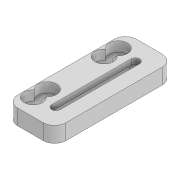
# Autodesk Inventor part: EStopHolder
Saved by Autodesk Inventor 2022 (Build 260153000, 153)
## iProperties
Created: 2022-11-15
Part Number: EStopHolder
Material: Generic
Document SubType Name: Modeling
Designer: MVeszpremi
Density: 1 g/cm^3
Appearance: Default
Author: MVeszpremi
Autodesk Inventor part; units mm, degrees
ref_plane "YZ Plane" through (0, 0, 0) normal (1, 0, 0) x (0, 1, 0)
ref_plane "XZ Plane" through (0, 0, 0) normal (0, 1, 0) x (-1, 0, 0)
ref_plane "XY Plane" through (0, 0, 0) normal (0, 0, 1) x (1, 0, 0)
sketch "Sketch1" plane through (0, 0, 0) normal (0, 1, 0) x (-1, 0, 0)
  line L0 (0, 0) -> (0, -28) construction
  line L1 (-1.5, 0) -> (-1.5, -28)
  line L2 (1.5, -28) -> (1.5, 0)
  arc A0 (1.5, 0) -> (-1.5, 0) centre (0, 0) ccw
  arc A1 (-1.5, -28) -> (1.5, -28) centre (0, -28) ccw
  line L3 (-6.5, 7) -> (10.5, 7)
  line L4 (10.5, 7) -> (10.5, -35)
  line L5 (10.5, -35) -> (-6.5, -35)
  line L6 (-6.5, -35) -> (-6.5, 7)
  line L7 (7, 7) -> (7, -35)
  circle A2 centre (7, -4) radius 1.5
  circle A3 centre (7, -24) radius 1.5
  line L8 (0, 1.5) -> (0, -29.5) construction
  line L9 (-3.5, 1.5) -> (-3.5, -29.5)
  line L10 (3.5, -29.5) -> (3.5, 1.5)
  arc A4 (3.5, 1.5) -> (-3.5, 1.5) centre (0, 1.5) ccw
  arc A5 (-3.5, -29.5) -> (3.5, -29.5) centre (0, -29.5) ccw
  circle A6 centre (7, 1) radius 1.5
  circle A7 centre (7, -29) radius 1.5
  point P0 (0, -14)
  point P1 (0, -14)
  dimension "d0" = 28
  dimension "d1" = 3
  dimension "d2" = 5
  dimension "d3" = 21
  dimension "d4" = 21
  dimension "d5" = 9
  dimension "d6" = 3.5
  dimension "d7" = 10
  dimension "d8" = 10
  dimension "d9" = 3
  dimension "d10" = 3
  dimension "d11" = 3.5
  dimension "d16" = 5
  dimension "d17" = 5
  dimension "d18" = 3
  dimension "d19" = 3
  constraints: 26 end point, 10 point on circle, 8 centre point, 8 tangent, 6 point on line, 4 parallel, 2 midpoint, 2 perpendicular, 1 horizontal, 1 vertical
  measures "d0" distance of L2.start L2.end
  measures "d1" distance between parallel lines of L1 L2
  measures "d2" distance between parallel lines of L6 L1
  measures "d3" distance from line of L3 point (0, -14)
  measures "d4" distance from line of point (0, -14) L5
  measures "d5" distance between parallel lines of L4 L2
  measures "d6" distance between parallel lines of L4 L7
  measures "d7" vertical distance of A2.centre point (0, -14)
  measures "d8" vertical distance of point (0, -14) A3.centre
  measures "d9" diameter of A2
  measures "d10" diameter of A3
  measures "d11" distance between parallel lines of L10 L0
  measures "d16" distance of A6.centre A2.centre
  measures "d17" distance of A3.centre A7.centre
  measures "d18" diameter of A7
  measures "d19" diameter of A6
extrude "Extrusion1" add sketch "Sketch1" along normal blind 5.5 contours L3 L7 A6 A2 A3 A7 L5 L6 | L3 L4 L5 L7 A7 A3 A2 A6 | A4 L10 A5 L9
extrude "Extrusion2" cut sketch "Sketch1" along normal blind 3.5 contours A4 L10 A5 L9
fillet "Fillet1" radius 4 4 edges at (-10.5, 2.75, 7) (-10.5, 2.75, -35) (6.5, 2.75, 7) (6.5, 2.75, -35)
sketch "Sketch2" plane through (0, 5.5, 0) normal (0, 1, 0) x (1, 0, 0)
  arc A0 (6.5, 31) -> (2.5, 35) centre (2.5, 31) ccw projected
  line L0 (2.5, 35) -> (-6.5, 35) projected
  arc A1 (-6.5, 35) -> (-10.5, 31) centre (-6.5, 31) ccw projected
  line L1 (-10.5, 31) -> (-10.5, -3) projected
  arc A2 (-10.5, -3) -> (-6.5, -7) centre (-6.5, -3) ccw projected
  line L2 (-6.5, -7) -> (2.5, -7) projected
  arc A3 (2.5, -7) -> (6.5, -3) centre (2.5, -3) ccw projected
  line L3 (6.5, -3) -> (6.5, 31) projected
  circle A4 centre (-7, -1) radius 1.5 projected
  circle A5 centre (-7, 4) radius 1.5 projected
  circle A6 centre (-7, 24) radius 1.5 projected
  circle A7 centre (-7, 29) radius 1.5 projected
  arc A8 (-1.5, 0) -> (1.5, 0) centre (0, 0) ccw projected
  line L4 (-1.5, 0) -> (-1.5, 28) projected
  arc A9 (1.5, 28) -> (-1.5, 28) centre (0, 28) ccw projected
  line L5 (1.5, 28) -> (1.5, 0) projected
  circle A10 centre (-7, -1) radius 3.25
  circle A11 centre (-7, 4) radius 3.25
  circle A12 centre (-7, 24) radius 3.25
  circle A13 centre (-7, 29) radius 3.25
  point P0 (-4.9233, 1.5)
  point P1 (-9.0767, 1.5)
  point P2 (-9.0767, 26.5)
  point P3 (-4.9233, 26.5)
  dimension "d21" = 6.5
  dimension "d22" = 6.5
  dimension "d23" = 6.5
  dimension "d24" = 6.5
  constraints: 4 centre point, 4 coincident
  measures "d21" diameter of A10
  measures "d22" diameter of A11
  measures "d23" diameter of A12
  measures "d24" diameter of A13
extrude "Extrusion3" cut sketch "Sketch2" against normal blind 3.5 contours A10 A11 | A11 A10 | A10 A11 | A12 A13 | A13 A12 | A12 A13
body "Solid1"
